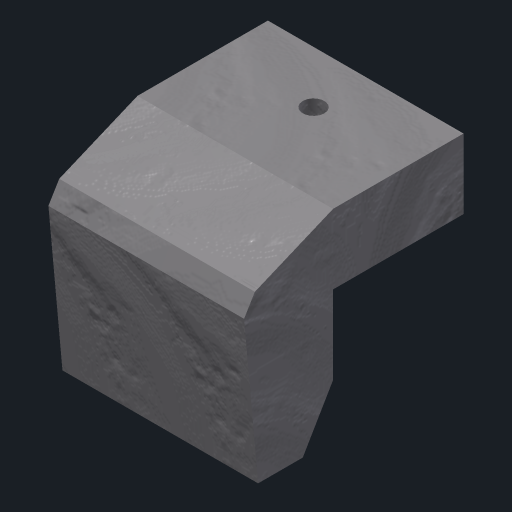
# Autodesk Inventor part: ESQUINA_RECTA_SUPERIOR
Saved by Autodesk Inventor 2024.3 (Build 283343000, 343)
## iProperties
Created: 2024-07-03
Part Number: ESQUINA_RECTA_SUPERIOR
Material: Steel, Mild, Welded
Document SubType Name: Modeling
Designer: Niler
Density: 7.85 g/cm^3
Appearance: Weld - Steel Mild
Author: Niler
Autodesk Inventor part; units mm, degrees
ref_plane "YZ Plane" through (0, 0, 0) normal (1, 0, 0) x (0, 1, 0)
ref_plane "XZ Plane" through (0, 0, 0) normal (0, 1, 0) x (-1, 0, 0)
sketch "Sketch1" plane through (0, 0, 0) normal (1, 0, 0) x (0, 1, 0)
  line L0 (0, 0) -> (10.7, 0)
  line L1 (10.7, 0) -> (10.7, -31.5)
  line L2 (10.7, -31.5) -> (0, -31.5)
  line L3 (0, -31.5) -> (0, 0)
  line L4 (0, 0) -> (-20, 0)
  line L5 (-20, 0) -> (-20, -11.5)
  line L6 (-20, -11.5) -> (0, -11.5)
  line L7 (0, -11.5) -> (0, 0)
  line L8 (-20, -6.8471) -> (-12.0113, -11.5)
  dimension "d0" = 10.7
  dimension "d1" = 11.5
  dimension "d2" = 20
  dimension "d4" = 20
  constraints: 18 end point, 4 parallel, 2 horizontal, 2 perpendicular, 2 point on line
  measures "d0" distance of L1.end L2.end
  measures "d1" distance of L5.end L4.end
  measures "d2" distance of L0.start L4.end
  measures "d4" distance between parallel lines of L2 L6
extrude "Extrusion1" add sketch "Sketch1" along normal blind 30 contours L0 L1 L2 L3 | L3 L6 L8 L5 L4
sketch "Sketch3" plane through (0, 0, -31.5) normal (0, -1, 0) x (1, 0, 0)
  line L0 (0, 20) -> (0, 0) projected
  line L1 (0, 0) -> (30, 0) projected
  line L2 (30, 20) -> (30, 0) projected
  line L3 (0, 20) -> (30, 20) projected
  circle A0 centre (15, 8) radius 1.65
  line L4 (15, 0) -> (15, 9.65)
  point P0 (0, 31.5)
  dimension "d10" = 3.3
  dimension "d11" = 8
  constraints: 2 end point, 1 centre point, 1 midpoint, 1 point on line, 1 vertical
  measures "d10" diameter of A0
  measures "d11" distance from line of L1 A0.centre
extrude "Extrusion3" cut sketch "Sketch3" against normal blind 40 contours A0 L4 | L4 A0
ref_plane "Work Plane1" through (0, 3, -31.5) normal (0, -1, 0) x (1, 0, 0)
sketch "Sketch4" plane through (0, 3, -31.5) normal (0, -1, 0) x (1, 0, 0)
  circle A0 centre (15, 8) radius 1.65 projected
  circle A1 centre (20, 8) radius 1.65 projected
  line L0 (15, 4.6514) -> (12.1, 6.3257)
  line L1 (12.1, 6.3257) -> (12.1, 9.6743)
  line L2 (12.1, 9.6743) -> (15, 11.3486)
  line L3 (15, 11.3486) -> (17.9, 9.6743)
  line L4 (17.9, 9.6743) -> (17.9, 6.3257)
  line L5 (17.9, 6.3257) -> (15, 4.6514)
  line L6 (17.9, 6.3257) -> (17.9, 0)
  line L7 (0, 0) -> (30, 0) projected
  line L8 (12.1, 6.3257) -> (12.1, 0)
  line L9 (17.9, 0) -> (12.1, 0)
  line L10 (0, 0) -> (30, 0) projected
  line L11 (15, 0) -> (15, 11.3486)
  circle A2 centre (15, 8) radius 1.65
  line L12 (15, 4.6514) -> (17.9, 6.3257)
  line L13 (17.9, 6.3257) -> (17.9, 9.6743)
  line L14 (17.9, 9.6743) -> (15, 11.3486)
  line L15 (15, 11.3486) -> (12.1, 9.6743)
  line L16 (12.1, 9.6743) -> (12.1, 6.3257)
  line L17 (12.1, 6.3257) -> (15, 4.6514)
  line L18 (12.1, 6.3257) -> (12.1, 0)
  line L19 (17.9, 6.3257) -> (17.9, 0)
  line L20 (12.1, 0) -> (17.9, 0)
  point P0 (0, 31.5)
  point P1 (40, 0)
  point P2 (12.1, 0)
  point P3 (17.9, 0)
  dimension "d16" = 5.8
  constraints: 38 end point, 10 symmetric about line, 2 coincident, 2 point on line, 2 vertical, 1 centre point, 1 collinear, 1 midpoint, 1 parallel, 1 vertical alignment, 14 other
  measures "d16" distance between parallel lines of L1 L4
extrude "Extrusion4" cut sketch "Sketch4" against normal blind 3 contours A0 L11 | A0 L11 L3 L4 L5 | L11 A0 | A0 L11 L0 L1 L2 | L11 L7 L8 L0 | L5 L6 L7 L11
sketch "Sketch5" plane through (0, 0, 0) normal (-1, 0, 0) x (0, 0, 1)
  line L0 (0, -20) -> (-6.8471, -20) projected
  line L1 (0, 10.7) -> (0, -20) projected
  line L2 (-31.5, 10.7) -> (0, 10.7) projected
  line L3 (-31.5, 0) -> (-31.5, 10.7) projected
  line L4 (-11.5, 0) -> (-31.5, 0) projected
  line L5 (-11.5, -12.0113) -> (-11.5, 0) projected
  line L6 (-6.8471, -20) -> (-11.5, -12.0113) projected
  line L7 (-11.5, 10.7) -> (2.3381, 4.9114)
  line L8 (2.3381, 4.9114) -> (0, -20)
  line L9 (-11.5, 0) -> (-11.5, 10.7)
  point P0 (0, 0)
  point P1 (0, 5.8894)
  dimension "d19" = 157.3
  dimension "d20" = 15
  constraints: 6 end point, 1 perpendicular, 1 point on line
  measures "d19" angle of L7 L2
  measures "d20" distance of L7.start L7.end
extrude "Extrusion5" add sketch "Sketch5" against normal up to surface (30 mm away) contours L1 L7 L8
chamfer "Chamfer1" distance 2 angle 45 1 edges at (15, 4.9114, 2.3381)
extrude "Extrusion6" cut sketch "Sketch5" against normal through all contours L7 L2 L1
body "Solid1"
